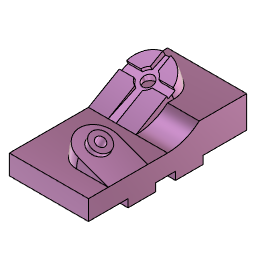
Exercise-10 v1 (Autodesk Fusion 360 design; units mm, degrees)
Autodesk Fusion 360 part; units mm, degrees
sketch "Sketch1" plane through (0, 0, 0) normal (1, 0, 0) x (0, 1, 0)
  line L0 (100, -12.5) -> (-100, -12.5)
  line L1 (-100, -12.5) -> (-100, 12.5)
  line L2 (-100, 12.5) -> (100, 12.5)
  line L3 (100, 12.5) -> (100, -12.5)
  line L4 (100, -12.5) -> (-100, 12.5) construction
  line L5 (-100, -12.5) -> (100, 12.5) construction
  line L6 (-50, -12.5) -> (-15, -12.5)
  line L7 (-15, -12.5) -> (-15, -22.5)
  line L8 (-15, -22.5) -> (-50, -22.5)
  line L9 (-50, -22.5) -> (-50, -12.5)
  line L10 (10, -12.5) -> (45, -12.5)
  line L11 (45, -12.5) -> (45, -22.5)
  line L12 (45, -22.5) -> (10, -22.5)
  line L13 (10, -22.5) -> (10, -12.5)
  line L14 (100, 12.5) -> (40, 12.5)
  line L15 (40, 12.5) -> (40, 27.5)
  line L16 (40, 27.5) -> (100, 27.5)
  line L17 (100, 27.5) -> (100, 12.5)
  arc A0 (0, 12.5) -> (40, 27.5) centre (0, 73.3333) ccw
  dimension "d1" = 200
  dimension "d2" = 25
  dimension "d3" = 35
  dimension "d4" = 10
  dimension "d5" = 35
  dimension "d6" = 10
  dimension "d7" = 60
  dimension "d8" = 15
  dimension "d9" = 50
  dimension "d10" = 25
  constraint horizontal L0
  constraint perpendicular L0 L1
  constraint parallel L0 L2
  constraint parallel L1 L3
  constraint coincident L4 origin
  constraint coincident L5 origin
  constraint horizontal L6
  constraint vertical L7
  constraint horizontal L8
  constraint vertical L9
  constraint coincident L0 L6.start
  constraint horizontal L10
  constraint vertical L11
  constraint horizontal L12
  constraint vertical L13
  constraint coincident L0 L10.start
  constraint horizontal L14
  constraint vertical L15
  constraint horizontal L16
  constraint vertical L17
  constraint tangent L2 A0
  constraint midpoint L2 A0.start
  measures "d1" distance of L1.end L2.end
  measures "d2" distance of L0.end L1.end
  measures "d3" distance of L6.start L6.end
  measures "d4" distance of L6.start L8.end
  measures "d5" distance of L10.start L10.end
  measures "d6" distance of L10.start L12.end
  measures "d7" distance of L2.end L14.end
  measures "d8" distance of L2.end L16.end
  measures "d9" distance of L1 L9
  measures "d10" distance of L7 L13
extrude "Extrude1" add sketch "Sketch1" along normal mid plane 100
sketch "Sketch2" plane through (0, 0, 12.5) normal (0, 0, 1) x (-1, 0, 0)
  line L0 (50, 100) -> (-50, 100)
  line L1 (-50, 100) -> (-50, 0)
  line L2 (-50, 0) -> (50, 0)
  line L3 (50, 0) -> (50, 100)
  circle A0 centre (-10, 50) radius 6
  circle A1 centre (-10, 50) radius 12.5
  circle A2 centre (-10, 50) radius 25
  line L4 (-10, 25) -> (-10, 75)
  line L5 (-10, 75) -> (-50, 75)
  line L6 (-50, 75) -> (-50, 25)
  line L7 (-50, 25) -> (-10, 25)
  circle A3 centre (20, -50) radius 7.5
  circle A4 centre (20, -50) radius 12.5
  circle A5 centre (20, -50) radius 30
  line L8 (50, -40) -> (50, -100)
  line L9 (50, -50) -> (-10, -50)
  line L10 (-10, -50) -> (-10, 0)
  line L11 (-10, 0) -> (50, 0)
  line L12 (50, 0) -> (50, -50)
  line L13 (-13.1018, -45) -> (53.1018, -45)
  line L14 (53.1018, -45) -> (53.1018, -55)
  line L15 (53.1018, -55) -> (-13.1018, -55)
  line L16 (-13.1018, -55) -> (-13.1018, -45)
  line L17 (-13.1018, -45) -> (53.1018, -55) construction
  line L18 (53.1018, -45) -> (-13.1018, -55) construction
  line L19 (15, 0) -> (25, 0)
  line L20 (25, 0) -> (25, -100)
  line L21 (25, -100) -> (15, -100)
  line L22 (15, -100) -> (15, 0)
  line L23 (15, 0) -> (25, -100) construction
  line L24 (25, 0) -> (15, -100) construction
  point P0 (20, -50)
  point P1 (20, -50)
  dimension "d13" = 12
  dimension "d14" = 25
  dimension "d15" = 50
  dimension "d16" = 50
  dimension "d17" = 40
  dimension "d26" = 15
  dimension "d27" = 25
  dimension "d28" = 60
  dimension "d29" = 50
  dimension "d30" = 10
  dimension "d31" = 10
  dimension "d32" = 100
  constraint concentric A0 A1
  constraint concentric A1 A2
  constraint perpendicular L4 L5
  constraint parallel L4 L6
  constraint parallel L5 L7
  constraint coincident A2 L4.end
  constraint vertical L4
  constraint coincident A2 L4.start
  constraint concentric A3 A4
  constraint concentric A3 A5
  constraint tangent A5 L8
  constraint perpendicular L9 L10
  constraint parallel L9 L11
  constraint parallel L10 L12
  constraint coincident A5 L9.end
  constraint perpendicular L8 L9
  constraint coincident A5 L9.start
  constraint horizontal L13
  constraint perpendicular L13 L14
  constraint parallel L13 L15
  constraint parallel L14 L16
  constraint coincident L17 P1
  constraint coincident L18 P1
  constraint coincident P1 P0
  constraint horizontal L19
  constraint perpendicular L19 L20
  constraint parallel L19 L21
  constraint parallel L20 L22
  constraint coincident L23 P1
  constraint coincident L24 P1
  measures "d13" diameter of A0
  measures "d14" diameter of A1
  measures "d15" diameter of A2
  measures "d16" distance of L0 A0.centre
  measures "d17" distance of L1 A0.centre
  measures "d26" diameter of A3
  measures "d27" diameter of A4
  measures "d28" diameter of A5
  measures "d29" distance of L2 P1
  measures "d30" distance of L13.end L14.end
  measures "d31" distance of L20.end L21.end
  measures "d32" distance of L19.end L20.end
revolve "Revolve1" add sketch "Sketch2" angle 20 about axis through (50, -100, 12.5) along (0, 1, 0) contours L1 A2 L5 L6 L7 | A1 A2 L4 | A1 A2 L4
revolve "Revolve2" add sketch "Sketch2" angle 30 about axis through (50, -100, 12.5) along (0, 1, 0) contours A0 A1 L4 | A0 A1 L4
revolve "Revolve3" add sketch "Sketch2" angle 30 about axis through (10, 0, 12.5) along (1, 0, 0) contours L2 A5 L8 L11 L12 L13 L20 | L2 A5 L10 L11 L13 L22 | A4 A5 L13 L20 | A4 A5 L13 L22 | A4 A5 L15 L20 | A4 A5 L15 L22
revolve "Revolve4" add sketch "Sketch2" angle 25 about axis through (10, 0, 12.5) along (1, 0, 0) contours L2 A5 L11 L19 L20 L22 | A4 A5 L20 L22 | A5 L8 L12 L13 | A4 A5 L9 L13 | A3 A4 L20 L22 | A3 A4 L13 L20 | A4 A5 L9 L15 | A5 L10 L13 | A4 A5 L9 L13 | A3 A4 L13 L22 | A3 A4 L9 L13 | A3 A4 L9 L15 | A4 A5 L9 L15 | A3 A4 L9 L13 | A4 A5 L20 L22 | A3 A4 L15 L20 | A3 A4 L9 L15 | A3 A4 L20 L22 | A3 A4 L15 L22
